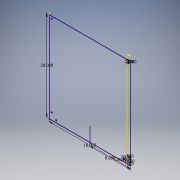
# Autodesk Inventor part: vrRig_v08_enclosure_backPanel
Saved by Autodesk Inventor 2016 (Build 200138000, 138)
## iProperties
Created: 2018-01-18
Part Number: vrRig_v08_enclosure_backPanel
Material: Generic
Document SubType Name: Modeling
Designer: harveylab
Density: 1 g/cm^3
Appearance: Default
Author: harveylab
Autodesk Inventor part; units mm, degrees
ref_plane "YZ Plane" through (0, 0, 0) normal (1, 0, 0) x (0, 1, 0)
ref_plane "XZ Plane" through (0, 0, 0) normal (0, 1, 0) x (-1, 0, 0)
ref_plane "XY Plane" through (0, 0, 0) normal (0, 0, 1) x (1, 0, 0)
ref_plane "Work Plane1" through (-6.5024, 0, 0) normal (0, 0, 1) x (1, 0, 0)
sketch "Sketch1" plane through (-6.5024, 0, 0) normal (0, 0, 1) x (1, 0, 0)
  line L0 (15.6512, -12.7) -> (15.6512, -25.4) projected
  line L1 (-440.9488, -12.7) -> (-440.9488, -25.4) projected
  line L2 (15.6512, -25.4) -> (-441.5488, -25.4)
  line L3 (-441.5488, -25.4) -> (-441.5488, -533.4)
  line L4 (-441.5488, -533.4) -> (15.6512, -533.4)
  line L5 (15.6512, -533.4) -> (15.6512, -25.4)
  line L6 (15.6512, -25.4) -> (2.9512, -25.4)
  line L7 (2.9512, -25.4) -> (2.9512, -38.1)
  circle A0 centre (2.9512, -38.1) radius 3.302
  line L8 (15.6512, -533.4) -> (15.6512, -495.3)
  line L9 (15.6512, -495.3) -> (2.9512, -495.3)
  circle A1 centre (2.9512, -495.3) radius 3.302
  line L10 (15.6512, -533.4) -> (15.6512, -520.7)
  line L11 (15.6512, -520.7) -> (-22.4488, -520.7)
  circle A2 centre (-22.4488, -520.7) radius 3.302
  line L12 (15.6512, -533.4) -> (-212.9488, -533.4)
  line L13 (-212.9488, -533.4) -> (-212.9488, -454.8045)
  circle A3 centre (-428.8488, -38.1) radius 3.302
  circle A4 centre (-428.8488, -495.3) radius 3.302
  circle A5 centre (-403.4488, -520.7) radius 3.302
  point P0 (6.5024, 0)
  dimension "d0" = 457.2
  dimension "d1" = 508
  dimension "d2" = 12.7
  dimension "d3" = 12.7
  dimension "d4" = 6.604
  dimension "d5" = 38.1
  dimension "d6" = 12.7
  dimension "d7" = 6.604
  dimension "d8" = 12.7
  dimension "d9" = 38.1
  dimension "d10" = 6.604
  dimension "d11" = 228.6
  constraints: 24 end point, 6 centre point, 5 perpendicular, 3 coincident, 3 point on line, 3 symmetric about line, 2 parallel, 1 horizontal, 1 midpoint, 3 other
  measures "d0" distance of L4.end L3.end
  measures "d1" distance of L3.end L2.end
  measures "d2" distance of L0.end L6.end
  measures "d3" distance of L6.end L7.end
  measures "d4" diameter of A0
  measures "d5" distance of L4.end L8.end
  measures "d6" distance of L8.end L9.end
  measures "d7" diameter of A1
  measures "d8" distance of L4.end L10.end
  measures "d9" distance of L10.end L11.end
  measures "d10" diameter of A2
  measures "d11" distance of L4.end L12.end
extrude "Extrusion1" add sketch "Sketch1" along normal blind 1.5875
body "Solid1"
